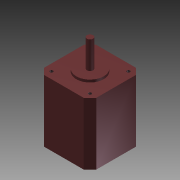
# Autodesk Inventor part: Motor
Saved by Autodesk Inventor 2012 SP1 (Build 160190100, 190)
## iProperties
Created: 2013-04-29
Part Number: Motor
Material: Default
Document SubType Name: Modeling
Designer: vogel
Density: 1 g/cm^3
Author: vogel
Autodesk Inventor part; units mm, degrees
ref_plane "YZ Plane" through (0, 0, 0) normal (1, 0, 0) x (0, 1, 0)
ref_plane "XZ Plane" through (0, 0, 0) normal (0, 1, 0) x (-1, 0, 0)
ref_plane "XY Plane" through (0, 0, 0) normal (0, 0, 1) x (1, 0, 0)
sketch "Skizze1" plane through (0, 0, 0) normal (0, 0, 1) x (1, 0, 0)
  line L0 (-21, 21) -> (21, 21)
  line L1 (21, 21) -> (21, -21)
  line L2 (21, -21) -> (-21, -21)
  line L3 (-21, -21) -> (-21, 21)
  line L4 (-29.4, 0) -> (29.4, 0) projected
  line L5 (0, -29.4) -> (0, 29.4) projected
  point P0 (0, 0)
  dimension "d0" = 42
  dimension "d1" = 42
  constraints: 8 end point, 2 parallel, 1 horizontal, 1 perpendicular, 2 other
  measures "d0" distance of L2.end L0.start
  measures "d1" distance between parallel lines of L1 L3
extrude "Extrusion1" add sketch "Skizze1" along normal blind 50
sketch "Skizze2" plane through (0, 0, 50) normal (0, 0, 1) x (1, 0, 0)
  circle A0 centre (0, 0) radius 11
  dimension "d4" = 22
  constraints: 1 centre point, 1 coincident
  measures "d4" diameter of A0
extrude "Extrusion2" add sketch "Skizze2" along normal blind 2
sketch "Skizze3" plane through (0, 0, 52) normal (0, 0, 1) x (1, 0, 0)
  circle A0 centre (0, 0) radius 11 projected
  circle A1 centre (0, 0) radius 2.5
  dimension "d7" = 5
  constraints: 1 centre point, 1 coincident
  measures "d7" diameter of A1
extrude "Extrusion3" add sketch "Skizze3" along normal blind 22 contours A1
chamfer "Fase1" distance 5 angle 45 4 edges at (-21, -21, 25) (21, -21, 25) (21, 21, 25) (-21, 21, 25)
sketch "Skizze4" plane through (0, 0, 50) normal (0, 0, 1) x (1, 0, 0)
  line L0 (-15.5, 15.5) -> (15.5, 15.5)
  line L1 (15.5, 15.5) -> (15.5, -15.5)
  line L2 (15.5, -15.5) -> (-15.5, -15.5)
  line L3 (-15.5, -15.5) -> (-15.5, 15.5)
  line L4 (-29.4, 0) -> (29.4, 0) projected
  line L5 (0, -29.4) -> (0, 29.4) projected
  dimension "d13" = 31
  constraints: 8 end point, 4 coincident, 2 parallel, 2 perpendicular, 1 horizontal, 2 other
  measures "d13" distance of L2.end L0.start
hole "Bohrung1" at (-15.5, 15.5, 50) at (15.5, 15.5, 50) at (15.5, -15.5, 50) at (-15.5, -15.5, 50) direction (0, 0, -1) diameter 2.459 depth 4.5 tip angle 118 thread size "M3x0.5" class "6H" standard "ISO Metric profile"
